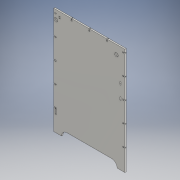
# Autodesk Inventor part: Højre side mk2
Saved by Autodesk Inventor 2016 (Build 200138000, 138)
## iProperties
Created: 2015-10-17
Part Number: Højre side mk2
Material: Generic
Document SubType Name: Modeling
Designer: iLyngklip
Density: 1 g/cm^3
Appearance: White
Author: iLyngklip
Autodesk Inventor part; units mm, degrees
ref_plane "YZ Plane" through (0, 0, 0) normal (1, 0, 0) x (0, 1, 0)
ref_plane "XZ Plane" through (0, 0, 0) normal (0, 1, 0) x (-1, 0, 0)
ref_plane "XY Plane" through (0, 0, 0) normal (0, 0, 1) x (1, 0, 0)
sketch "Sketch1" plane through (0, 0, 0) normal (0, 1, 0) x (-1, 0, 0)
  line L0 (160, 240) -> (-160, 240)
  line L1 (-160, 240) -> (-160, -240)
  line L2 (-160, -240) -> (160, -240)
  line L3 (160, -240) -> (160, 240)
  point P0 (0, 0)
  dimension "d0" = 320
  dimension "d1" = 480
  dimension "d2" = 240
  dimension "d3" = 160
  constraints: 8 end point, 2 parallel, 1 horizontal, 1 perpendicular
  measures "d0" distance of L1.end L2.end
  measures "d1" distance of L2.end L0.start
  measures "d2" distance from line of point (0, 0) L0
  measures "d3" distance from line of point (0, 0) L3
extrude "Tykkelse" add sketch "Sketch1" along normal blind 6
sketch "Sketch2" plane through (0, 6, 0) normal (0, 1, 0) x (1, 0, 0)
  line L0 (160, 240) -> (-160, 240) construction
  arc A0 (100, 215) -> (125, 240) centre (100, 240) ccw
  arc A1 (-125, 240) -> (-100, 215) centre (-100, 240) ccw
  line L1 (-100, 215) -> (100, 215)
  line L2 (-125, 240) -> (125, 240)
  point P0 (0, 0)
  dimension "d6" = 50
  dimension "d7" = 50
  dimension "d8" = 60
  dimension "d9" = 60
  constraints: 4 end point, 4 point on circle, 4 point on line, 2 centre point, 1 collinear, 1 horizontal, 1 tangent
  measures "d6" diameter of A0
  measures "d7" diameter of A1
  measures "d8" distance of L0.start A0.centre
  measures "d9" distance of A1.centre L0.end
extrude "Fødder" cut sketch "Sketch2" against normal up to surface (6 mm away)
sketch "Sketch4" plane through (0, 0, 0) normal (0, -1, 0) x (1, 0, 0)
  arc A0 (-100, -215) -> (-125, -240) centre (-100, -240) ccw construction
  line L0 (-100, -215) -> (100, -215) construction
  arc A1 (125, -240) -> (100, -215) centre (100, -240) ccw construction
  line L1 (160, -240) -> (125, -240) construction
  line L2 (160, 240) -> (160, -240) construction
  line L3 (-160, 240) -> (160, 240) construction
  line L4 (-160, -240) -> (-160, 240) construction
  line L5 (-125, -240) -> (-160, -240) construction
  line L6 (160, 240) -> (160, -240) projected
  line L7 (160, 240) -> (160, -240) projected
  line L8 (160, -142.5) -> (153.679, -142.5)
  line L9 (150.8, -141.25) -> (152.2, -141.25)
  line L10 (152.2, -146.75) -> (150.8, -146.75)
  arc A2 (149.302, -145.3277) -> (150.8, -146.75) centre (150.8, -145.25) ccw
  arc A3 (150.8, -141.25) -> (149.302, -142.6723) centre (150.8, -142.75) ccw
  arc A4 (149.302, -142.6723) -> (149.302, -145.3277) centre (150, -144) ccw
  arc A5 (153.679, -142.5) -> (152.2, -141.25) centre (152.2, -142.75) ccw
  line L11 (160, -145.5) -> (153.679, -145.5)
  arc A6 (152.2, -146.75) -> (153.679, -145.5) centre (152.2, -145.25) ccw
  line L12 (150, -144) -> (160, -144) construction
  arc A7 (149.302, -50.6723) -> (149.302, -53.3277) centre (150, -52) ccw
  arc A8 (149.302, -53.3277) -> (150.8, -54.75) centre (150.8, -53.25) ccw
  line L13 (152.2, -54.75) -> (150.8, -54.75)
  arc A9 (150.8, -49.25) -> (149.302, -50.6723) centre (150.8, -50.75) ccw
  line L14 (150.8, -49.25) -> (152.2, -49.25)
  arc A10 (152.2, -54.75) -> (153.679, -53.5) centre (152.2, -53.25) ccw
  arc A11 (153.679, -50.5) -> (152.2, -49.25) centre (152.2, -50.75) ccw
  line L15 (160, -53.5) -> (153.679, -53.5)
  line L16 (150, -52) -> (160, -52) construction
  line L17 (160, -50.5) -> (153.679, -50.5)
  arc A12 (149.302, 41.3277) -> (149.302, 38.6723) centre (150, 40) ccw
  arc A13 (149.302, 38.6723) -> (150.8, 37.25) centre (150.8, 38.75) ccw
  line L18 (152.2, 37.25) -> (150.8, 37.25)
  arc A14 (150.8, 42.75) -> (149.302, 41.3277) centre (150.8, 41.25) ccw
  line L19 (150.8, 42.75) -> (152.2, 42.75)
  arc A15 (152.2, 37.25) -> (153.679, 38.5) centre (152.2, 38.75) ccw
  arc A16 (153.679, 41.5) -> (152.2, 42.75) centre (152.2, 41.25) ccw
  line L20 (160, 38.5) -> (153.679, 38.5)
  line L21 (150, 40) -> (160, 40) construction
  line L22 (160, 41.5) -> (153.679, 41.5)
  arc A17 (149.302, 133.3277) -> (149.302, 130.6723) centre (150, 132) ccw
  arc A18 (149.302, 130.6723) -> (150.8, 129.25) centre (150.8, 130.75) ccw
  line L23 (152.2, 129.25) -> (150.8, 129.25)
  arc A19 (150.8, 134.75) -> (149.302, 133.3277) centre (150.8, 133.25) ccw
  line L24 (150.8, 134.75) -> (152.2, 134.75)
  arc A20 (152.2, 129.25) -> (153.679, 130.5) centre (152.2, 130.75) ccw
  arc A21 (153.679, 133.5) -> (152.2, 134.75) centre (152.2, 133.25) ccw
  line L25 (160, 130.5) -> (153.679, 130.5)
  line L26 (150, 132) -> (160, 132) construction
  line L27 (160, 133.5) -> (153.679, 133.5)
  arc A22 (149.302, 225.3277) -> (149.302, 222.6723) centre (150, 224) ccw
  arc A23 (149.302, 222.6723) -> (150.8, 221.25) centre (150.8, 222.75) ccw
  line L28 (152.2, 221.25) -> (150.8, 221.25)
  arc A24 (150.8, 226.75) -> (149.302, 225.3277) centre (150.8, 225.25) ccw
  line L29 (150.8, 226.75) -> (152.2, 226.75)
  arc A25 (152.2, 221.25) -> (153.679, 222.5) centre (152.2, 222.75) ccw
  arc A26 (153.679, 225.5) -> (152.2, 226.75) centre (152.2, 225.25) ccw
  line L30 (160, 222.5) -> (153.679, 222.5)
  line L31 (150, 224) -> (160, 224) construction
  line L32 (160, 225.5) -> (153.679, 225.5)
  line L33 (0, -5.1965) -> (0, 140.9006) construction
  line L34 (-160, -142.5) -> (-153.679, -142.5)
  line L35 (-150.8, -141.25) -> (-152.2, -141.25)
  line L36 (-152.2, -146.75) -> (-150.8, -146.75)
  arc A27 (-150.8, -146.75) -> (-149.302, -145.3277) centre (-150.8, -145.25) ccw
  arc A28 (-149.302, -142.6723) -> (-150.8, -141.25) centre (-150.8, -142.75) ccw
  arc A29 (-149.302, -145.3277) -> (-149.302, -142.6723) centre (-150, -144) ccw
  arc A30 (-152.2, -141.25) -> (-153.679, -142.5) centre (-152.2, -142.75) ccw
  line L37 (-160, -145.5) -> (-153.679, -145.5)
  arc A31 (-153.679, -145.5) -> (-152.2, -146.75) centre (-152.2, -145.25) ccw
  line L38 (-150, -144) -> (-160, -144) construction
  arc A32 (-149.302, -53.3277) -> (-149.302, -50.6723) centre (-150, -52) ccw
  arc A33 (-150.8, -54.75) -> (-149.302, -53.3277) centre (-150.8, -53.25) ccw
  line L39 (-152.2, -54.75) -> (-150.8, -54.75)
  arc A34 (-149.302, -50.6723) -> (-150.8, -49.25) centre (-150.8, -50.75) ccw
  line L40 (-150.8, -49.25) -> (-152.2, -49.25)
  arc A35 (-153.679, -53.5) -> (-152.2, -54.75) centre (-152.2, -53.25) ccw
  arc A36 (-152.2, -49.25) -> (-153.679, -50.5) centre (-152.2, -50.75) ccw
  line L41 (-160, -53.5) -> (-153.679, -53.5)
  line L42 (-150, -52) -> (-160, -52) construction
  line L43 (-160, -50.5) -> (-153.679, -50.5)
  arc A37 (-149.302, 38.6723) -> (-149.302, 41.3277) centre (-150, 40) ccw
  arc A38 (-150.8, 37.25) -> (-149.302, 38.6723) centre (-150.8, 38.75) ccw
  line L44 (-152.2, 37.25) -> (-150.8, 37.25)
  arc A39 (-149.302, 41.3277) -> (-150.8, 42.75) centre (-150.8, 41.25) ccw
  line L45 (-150.8, 42.75) -> (-152.2, 42.75)
  arc A40 (-153.679, 38.5) -> (-152.2, 37.25) centre (-152.2, 38.75) ccw
  arc A41 (-152.2, 42.75) -> (-153.679, 41.5) centre (-152.2, 41.25) ccw
  line L46 (-160, 38.5) -> (-153.679, 38.5)
  line L47 (-150, 40) -> (-160, 40) construction
  line L48 (-160, 41.5) -> (-153.679, 41.5)
  arc A42 (-149.302, 130.6723) -> (-149.302, 133.3277) centre (-150, 132) ccw
  arc A43 (-150.8, 129.25) -> (-149.302, 130.6723) centre (-150.8, 130.75) ccw
  line L49 (-152.2, 129.25) -> (-150.8, 129.25)
  arc A44 (-149.302, 133.3277) -> (-150.8, 134.75) centre (-150.8, 133.25) ccw
  line L50 (-150.8, 134.75) -> (-152.2, 134.75)
  arc A45 (-153.679, 130.5) -> (-152.2, 129.25) centre (-152.2, 130.75) ccw
  arc A46 (-152.2, 134.75) -> (-153.679, 133.5) centre (-152.2, 133.25) ccw
  line L51 (-160, 130.5) -> (-153.679, 130.5)
  line L52 (-150, 132) -> (-160, 132) construction
  line L53 (-160, 133.5) -> (-153.679, 133.5)
  arc A47 (-149.302, 222.6723) -> (-149.302, 225.3277) centre (-150, 224) ccw
  arc A48 (-150.8, 221.25) -> (-149.302, 222.6723) centre (-150.8, 222.75) ccw
  line L54 (-152.2, 221.25) -> (-150.8, 221.25)
  arc A49 (-149.302, 225.3277) -> (-150.8, 226.75) centre (-150.8, 225.25) ccw
  line L55 (-150.8, 226.75) -> (-152.2, 226.75)
  arc A50 (-153.679, 222.5) -> (-152.2, 221.25) centre (-152.2, 222.75) ccw
  arc A51 (-152.2, 226.75) -> (-153.679, 225.5) centre (-152.2, 225.25) ccw
  line L56 (-160, 222.5) -> (-153.679, 222.5)
  line L57 (-150, 224) -> (-160, 224) construction
  line L58 (-160, 225.5) -> (-153.679, 225.5)
  line L59 (-81.5, 240) -> (-81.5, 233.679)
  line L60 (-82.75, 230.8) -> (-82.75, 232.2)
  line L61 (-77.25, 232.2) -> (-77.25, 230.8)
  arc A52 (-78.6723, 229.302) -> (-77.25, 230.8) centre (-78.75, 230.8) ccw
  arc A53 (-82.75, 230.8) -> (-81.3277, 229.302) centre (-81.25, 230.8) ccw
  arc A54 (-81.3277, 229.302) -> (-78.6723, 229.302) centre (-80, 230) ccw
  arc A55 (-81.5, 233.679) -> (-82.75, 232.2) centre (-81.25, 232.2) ccw
  line L62 (-78.5, 240) -> (-78.5, 233.679)
  arc A56 (-77.25, 232.2) -> (-78.5, 233.679) centre (-78.75, 232.2) ccw
  line L63 (-160, 240) -> (160, 240) projected
  line L64 (-80, 230) -> (-80, 240) construction
  line L65 (2.75, 232.2) -> (2.75, 230.8)
  arc A57 (2.75, 232.2) -> (1.5, 233.679) centre (1.25, 232.2) ccw
  arc A58 (1.3277, 229.302) -> (2.75, 230.8) centre (1.25, 230.8) ccw
  line L66 (1.5, 240) -> (1.5, 233.679)
  line L67 (0, 230) -> (0, 240) construction
  line L68 (-1.5, 240) -> (-1.5, 233.679)
  arc A59 (-2.75, 230.8) -> (-1.3277, 229.302) centre (-1.25, 230.8) ccw
  line L69 (-2.75, 230.8) -> (-2.75, 232.2)
  arc A60 (-1.5, 233.679) -> (-2.75, 232.2) centre (-1.25, 232.2) ccw
  arc A61 (-1.3277, 229.302) -> (1.3277, 229.302) centre (0, 230) ccw
  line L70 (82.75, 232.2) -> (82.75, 230.8)
  arc A62 (82.75, 232.2) -> (81.5, 233.679) centre (81.25, 232.2) ccw
  arc A63 (81.3277, 229.302) -> (82.75, 230.8) centre (81.25, 230.8) ccw
  line L71 (81.5, 240) -> (81.5, 233.679)
  line L72 (80, 230) -> (80, 240) construction
  line L73 (78.5, 240) -> (78.5, 233.679)
  arc A64 (77.25, 230.8) -> (78.6723, 229.302) centre (78.75, 230.8) ccw
  line L74 (77.25, 230.8) -> (77.25, 232.2)
  arc A65 (78.5, 233.679) -> (77.25, 232.2) centre (78.75, 232.2) ccw
  arc A66 (78.6723, 229.302) -> (81.3277, 229.302) centre (80, 230) ccw
  line L75 (-160, 222.5) -> (-160, 225.5)
  line L76 (-160, 130.5) -> (-160, 133.5)
  line L77 (-160, 41.5) -> (-160, 38.5)
  line L78 (-160, -240) -> (-160, 240) projected
  line L79 (-160, -50.5) -> (-160, -53.5)
  line L80 (-160, -142.5) -> (-160, -145.5)
  line L81 (160, -50.5) -> (160, -53.5)
  line L82 (160, 38.5) -> (160, 41.5)
  line L83 (160, 130.5) -> (160, 133.5)
  line L84 (160, 222.5) -> (160, 225.5)
  line L85 (81.5, 240) -> (78.5, 240)
  line L86 (-160, 240) -> (160, 240) projected
  line L87 (1.5, 240) -> (-1.5, 240)
  line L88 (-78.5, 240) -> (-81.5, 240)
  dimension "d284" = 1.4
  dimension "d285" = 2.5
  dimension "d286" = 10
  dimension "d287" = 1.5
  dimension "d290" = 0.25
  dimension "d291" = 7.8
  dimension "d292" = 3
  dimension "d293" = 1.5
  dimension "d294" = 1.5
  dimension "d295" = 1.5
  dimension "d296" = 1.5
  dimension "d297" = 1.5
  dimension "d298" = 96
  dimension "d301" = 92
  dimension "d306" = 464
  dimension "d307" = 372
  dimension "d308" = 188
  dimension "d309" = 280
  dimension "d310" = 160
  dimension "d311" = 160
  dimension "d312" = 0
  dimension "d313" = 2.5
  dimension "d314" = 1.5
  dimension "d315" = 0.25
  dimension "d316" = 3
  dimension "d317" = 1.5
  dimension "d318" = 1.5
  dimension "d319" = 1.5
  dimension "d320" = 1.5
  dimension "d321" = 1.5
  dimension "d323" = 10
  dimension "d324" = 7.8
  dimension "d325" = 1.4
  dimension "d326" = 80
  dimension "d329" = 80
  constraints: 156 end point, 130 point on circle, 80 symmetric about line, 65 centre point, 10 collinear, 9 vertical, 5 horizontal alignment, 5 point on line, 4 horizontal, 4 tangent, 3 vertical alignment, 2 perpendicular, 181 other
  measures "d284" distance of A5.centre A3.centre
  measures "d285" distance of A5.centre A6.centre
  measures "d286" distance from line of L2 L12.start
  measures "d287" distance from line of L12.start L8
  measures "d290" distance from line of L8 A5.centre
  measures "d291" distance from line of L2 A5.centre
  measures "d292" distance between parallel lines of L11 L8
  measures "d293" radius of A4
  measures "d294" radius of A3
  measures "d295" radius of A5
  measures "d296" radius of A6
  measures "d297" radius of A2
  measures "d298" distance between parallel lines of L1 L12
  measures "d301" distance of A2.start A7.end
  measures "d306" distance between parallel lines of L1 L31
  measures "d307" distance between parallel lines of L1 L26
  measures "d308" distance between parallel lines of L1 L16
  measures "d309" distance between parallel lines of L1 L21
  measures "d310" distance between parallel lines of L2 L33
  measures "d311" distance between parallel lines of L4 L33
  measures "d312" horizontal distance of A55.centre A53.centre
  measures "d313" distance of A55.centre A56.centre
  measures "d314" distance from line of L64.start L59
  measures "d315" distance from line of L59 A55.centre
  measures "d316" distance between parallel lines of L62 L59
  measures "d317" radius of A54
  measures "d318" radius of A53
  measures "d319" radius of A55
  measures "d320" radius of A56
  measures "d321" radius of A52
  measures "d323" vertical distance of L62.start L64.start
  measures "d324" vertical distance of L62.start A56.centre
  measures "d325" distance of A55.centre A53.centre
  measures "d326" distance between parallel lines of L4 L64
  measures "d329" distance of L61.end L65.end
mirror "Mirror1" about plane through (0, 6, 0) normal (0, 1, 0) remove original yes
sketch "Sketch6" plane through (0, 6, 0) normal (0, 1, 0) x (1, 0, 0)
  circle A0 centre (122, -200) radius 4 construction
  line L0 (160, -240) -> (160, 240) projected
  circle A1 centre (-150, -200) radius 4 construction
  line L1 (-160, -240) -> (160, -240) projected
  line L2 (-160, 240) -> (-160, -240) projected
  circle A2 centre (-150, -200) radius 4 construction
  circle A3 centre (-150, -200) radius 8
  circle A4 centre (122, -200) radius 8
  line L3 (160, -240) -> (160, 240) projected
  point P0 (0, 0)
  point P1 (160, -221.75)
  point P2 (-160, -129.75)
  point P3 (-160, -218.25)
  point P4 (160, -218.25)
  point P5 (160, -129.75)
  dimension "d140" = 8
  dimension "d154" = 8
  dimension "d155" = 40
  dimension "d170" = 10
  dimension "d174" = 40
  dimension "d233" = 16
  dimension "d234" = 16
  dimension "d235" = 38
  constraints: 5 centre point, 4 coincident, 1 concentric
  measures "d140" diameter of A0
  measures "d154" diameter of A1
  measures "d155" distance from line of L1 A1.centre
  measures "d170" distance from line of L2 A1.centre
  measures "d174" distance from line of L1 A0.centre
  measures "d233" diameter of A3
  measures "d234" diameter of A4
  measures "d235" distance from line of L3 A0.centre
sketch "Sketch7" plane through (-160, 12, 240) normal (0, 1, 0) x (1, 0, 0)
  circle A0 centre (300, 202) radius 2.5 construction
  circle A1 centre (300, 142) radius 2.5 construction
  line L0 (320, 0) -> (320, 480) projected
  line L1 (0, 0) -> (320, 0) projected
  arc A2 (297.5, 137) -> (302.5, 137) centre (300, 137) ccw
  arc A3 (302.5, 207) -> (297.5, 207) centre (300, 207) ccw
  arc A4 (297.5, 197) -> (302.5, 197) centre (300, 197) ccw
  line L2 (300, 207) -> (300, 137) construction
  arc A5 (302.5, 147) -> (297.5, 147) centre (300, 147) ccw
  line L3 (302.5, 207) -> (302.5, 197)
  line L4 (297.5, 197) -> (297.5, 207)
  line L5 (297.5, 147) -> (297.5, 137)
  line L6 (302.5, 137) -> (302.5, 147)
  point P0 (160, 240)
  point P1 (320, 21.75)
  point P2 (320, 110.25)
  dimension "d180" = 20
  dimension "d182" = 202
  dimension "d184" = 60
  dimension "d185" = 5
  dimension "d186" = 5
  dimension "d190" = 5
  dimension "d191" = 5
  dimension "d192" = 5
  dimension "d193" = 5
  dimension "d194" = 5
  dimension "d195" = 10
  dimension "d196" = 5
  dimension "d197" = 10
  constraints: 10 end point, 8 point on circle, 8 tangent, 6 centre point, 4 point on line, 1 vertical
  measures "d180" distance from line of L0 A0.centre
  measures "d182" distance from line of L1 A0.centre
  measures "d184" distance of A1.centre A0.centre
  measures "d185" diameter of A1
  measures "d186" diameter of A0
  measures "d190" diameter of A3
  measures "d191" diameter of A4
  measures "d192" diameter of A2
  measures "d193" diameter of A5
  measures "d194" distance of L2.end A1.centre
  measures "d195" distance of L2.end A5.centre
  measures "d196" distance of A0.centre A4.centre
  measures "d197" distance of A4.centre L2.start
extrude "Motor Monterings huller" cut sketch "Sketch7" against normal up to surface (6 mm away)
extrude "Leje hul" cut sketch "Sketch6" along normal blind 3.5
sketch "Sketch8" plane through (-160, 12, 240) normal (0, 1, 0) x (1, 0, 0)
  line L0 (23, 20) -> (29, 20) construction
  arc A0 (29, 19) -> (29, 21) centre (29, 20) ccw
  arc A1 (23, 21) -> (23, 19) centre (23, 20) ccw
  line L1 (23, 21) -> (29, 21)
  line L2 (29, 19) -> (23, 19)
  line L3 (23, 26.5) -> (29, 26.5) construction
  arc A2 (29, 25.5) -> (29, 27.5) centre (29, 26.5) ccw
  arc A3 (23, 27.5) -> (23, 25.5) centre (23, 26.5) ccw
  line L4 (23, 27.5) -> (29, 27.5)
  line L5 (23, 25.5) -> (29, 25.5)
  line L6 (0, 0) -> (320, 0) projected
  line L7 (0, 480) -> (0, 0) projected
  point P0 (160, 240)
  dimension "d243" = 2
  dimension "d244" = 2
  dimension "d245" = 6
  dimension "d247" = 2
  dimension "d248" = 2
  dimension "d249" = 6
  dimension "d336" = 6.5
  dimension "d337" = 20
  dimension "d338" = 23
  constraints: 14 end point, 8 point on circle, 7 tangent, 4 centre point, 3 horizontal, 2 coincident, 1 vertical alignment
  measures "d243" diameter of A1
  measures "d244" diameter of A0
  measures "d245" distance of L0.start L0.end
  measures "d247" diameter of A3
  measures "d248" diameter of A2
  measures "d249" distance of L3.end L3.start
  measures "d336" distance between parallel lines of L0 L3
  measures "d337" distance between parallel lines of L6 L0
  measures "d338" distance from line of L7 L0.start
extrude "Endstop hul" cut sketch "Sketch8" against normal blind 10
extrude "Monteringshuller" cut sketch "Sketch4" against normal blind 11
sketch "Sketch9" plane through (-100, 6, -215) normal (0, -1, 0) x (1, 0, 0)
  line L0 (-52.46, 66.5) -> (-49.46, 66.5) construction
  line L1 (-49.46, 66.5) -> (-49.46, 46.5) construction
  line L2 (-49.46, 46.5) -> (-52.46, 46.5) construction
  line L3 (-52.46, 46.5) -> (-52.46, 66.5) construction
  line L4 (-48.46, 45.5) -> (-48.46, 67.5)
  line L5 (-48.46, 67.5) -> (-53.46, 67.5)
  line L6 (-53.46, 67.5) -> (-53.46, 45.5)
  line L7 (-53.46, 45.5) -> (-48.46, 45.5)
  point P0 (100, 215)
  dimension "d339" = 1
  constraints: 8 end point, 3 other
  measures "d339" distance between parallel lines of L1 L4
extrude "SD-kort hul" cut sketch "Sketch9" against normal up to next
fillet "SD-kort" radius 1.5 4 edges at (-153.46, 9, -147.5) (-148.46, 9, -147.5) (-148.46, 9, -169.5) (-153.46, 9, -169.5)
equation "\"d2\" = 0.5 * d1"
equation "\"d3\" = 0.5 * d0"
equation "\"d6\" = d7"
equation "\"d9\" = d8"
body "Solid1"
